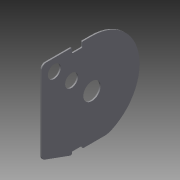
# Autodesk Inventor part: InnerFlange27130914
Saved by Autodesk Inventor 2015 (Build 190159000, 159)
## iProperties
Created: 2014-06-27
Part Number: InnerFlange27130914
Material: Generic
Document SubType Name: Modeling
Designer: STACKPOLE
Density: 1 g/cm^3
Appearance: Default
Author: STACKPOLE
Autodesk Inventor part; units mm, degrees
ref_plane "YZ Plane" through (0, 0, 0) normal (1, 0, 0) x (0, 1, 0)
ref_plane "XZ Plane" through (0, 0, 0) normal (0, 1, 0) x (-1, 0, 0)
ref_plane "XY Plane" through (0, 0, 0) normal (0, 0, 1) x (1, 0, 0)
sketch "Sketch1" plane through (0, 0, 0) normal (1, 0, 0) x (0, 1, 0)
  line L0 (-58, -40) -> (-58, 50)
  line L1 (0, 0) -> (-57.3223, 54.5531) construction
  circle A0 centre (-23.5426, 22.4053) radius 7.5
  circle A1 centre (0, 0) radius 47 construction
  circle A2 centre (-43.4633, 41.3636) radius 7.5
  circle A3 centre (0, 0) radius 10
  line L2 (-11, -52) -> (14.1774, -52)
  line L3 (-58, 0) -> (-58, -40)
  line L4 (0, 0) -> (0, -52) construction
  line L5 (-58, -40) -> (-23, -52.739)
  circle A4 centre (0, 0) radius 50 construction
  arc A5 (22.2788, -50.2857) -> (0, 55) centre (0, 0) ccw
  line L6 (-43.4633, 41.3636) -> (-48.6337, 35.9307)
  arc A6 (-53, 55) -> (-58, 50) centre (-53, 50) ccw
  line L7 (-11, 54) -> (-11, 50)
  line L8 (-12, 49) -> (-22, 49)
  line L9 (-23, 50) -> (-23, 54)
  line L10 (-53, 55) -> (-24, 55)
  line L11 (-10, 55) -> (0, 55)
  arc A7 (-23, 54) -> (-24, 55) centre (-24, 54) ccw
  arc A8 (-10, 55) -> (-11, 54) centre (-10, 54) ccw
  arc A9 (-12, 49) -> (-11, 50) centre (-12, 50) ccw
  arc A10 (-23, 50) -> (-22, 49) centre (-22, 50) ccw
  arc A11 (14.1774, -52) -> (22.2788, -50.2857) centre (14.1774, -32) ccw
  line L12 (-23, -49.5) -> (-23, -52.739)
  line L13 (-11, -52) -> (-11, -49.5)
  line L14 (-11.5, -49) -> (-22.5, -49)
  arc A12 (-11, -49.5) -> (-11.5, -49) centre (-11.5, -49.5) ccw
  arc A13 (-22.5, -49) -> (-23, -49.5) centre (-22.5, -49.5) ccw
  point P0 (-28.9755, 27.5757)
  point P1 (-57.7919, 55)
  point P2 (-58, 55)
  point P3 (-25.2108, 39.6663)
  point P4 (17.9165, -52)
  point P5 (-23, 55)
  point P6 (-11, 52)
  dimension "d4" = 94
  dimension "d6" = 15
  dimension "d7" = 15
  dimension "d3" = 32.5
  dimension "d8" = 60
  dimension "d9" = 20
  dimension "d13" = 52
  dimension "d20" = 100
  dimension "d31" = 55
  dimension "d34" = 58
  dimension "d52" = 5
  dimension "d54" = 47
  dimension "d56" = 1
  dimension "d59" = 20
  dimension "d60" = 12
  dimension "d61" = 6
  dimension "d65" = 0.5
  dimension "d69" = 95
  dimension "d72" = 110
  dimension "d73" = 3
  dimension "d74" = 12
  constraints: 30 end point, 19 point on circle, 17 tangent, 11 centre point, 11 point on line, 4 coincident, 4 equal radius, 4 perpendicular, 3 vertical, 2 horizontal, 1 midpoint, 1 parallel, 1 vertical alignment, 9 other
  measures "d3" distance of point (0, 0) point (-23.543, 22.405)
  measures "d8" distance of point (0, 0) L6.start
  measures "d9" diameter of A3
  measures "d13" distance from line of L2 L4.start
  measures "d20" diameter of A4
  measures "d31" radius of A5
  measures "d34" distance from line of point (0, 0) L0
  measures "d52" radius of A6
  measures "d54" distance between parallel lines of L0 L7
  measures "d56" radius of A7
  measures "d59" radius of A11
  measures "d60" distance between parallel lines of L9 L7
  measures "d61" distance between parallel lines of L8 L10
  measures "d65" radius of A12
  measures "d69" distance from line of L0.start L10
  measures "d72" angle of L5 L0
  measures "d73" distance between parallel lines of L2 L14
  measures "d74" distance between parallel lines of L13 L12
extrude "Extrusion3" add sketch "Sketch1" along normal blind 1.5
fillet "Fillet1" radius 5 1 edges at (0.75, -58, -40)
fillet "Fillet2" radius 1.5 2 edges at (0.75, -23, -52.739) (0.75, -11, -52)
body "Solid3"
